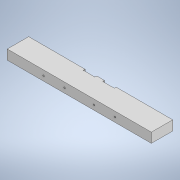
# Autodesk Inventor part: caster_wheel_mount
Saved by Autodesk Inventor 2020 (Build 240168000, 168)
## iProperties
Created: 2022-06-22
Part Number: caster_wheel_mount
Material: 일반
Document SubType Name: Modeling
Designer: samsung
Density: 1 g/cm^3
Appearance: 기본값
Author: samsung
Autodesk Inventor part; units mm, degrees
ref_plane "YZ Plane" through (0, 0, 0) normal (1, 0, 0) x (0, 1, 0)
ref_plane "작업 평면1" through (-15, 261.5, -15) normal (0, 1, 0) x (-1, 0, 0)
ref_plane "작업 평면4" through (-15, 241.5, -15) normal (0, 1, 0) x (1, 0, 0)
sketch "스케치4" plane through (-15, 241.5, -15) normal (0, 1, 0) x (1, 0, 0)
  line L0 (15, -15) -> (15, -10.3) projected
  line L1 (-15, -15) -> (15, -15) projected
  line L2 (-15, -10.3) -> (-15, -15) projected
  line L3 (-35, -10.3) -> (-15, -10.3) projected
  line L4 (-35, -15) -> (-35, -10.3) projected
  line L5 (-65, -15) -> (-35, -15) projected
  line L6 (-65, -10.3) -> (-65, -15) projected
  line L7 (-101.5, -10.3) -> (-65, -10.3) projected
  line L8 (51.5, -65.3) -> (-101.5, -65.3) projected
  line L9 (15, -10.3) -> (51.5, -10.3) projected
  line L10 (-105, -65.3) -> (-105, -10.3)
  line L11 (55, -65.3) -> (55, -10.3)
  line L12 (-105, -65.3) -> (55, -65.3)
  line L13 (-101.5, -10.3) -> (-65, -10.3) projected
  line L14 (-105, -10.3) -> (-65, -10.3)
  line L15 (55, -10.3) -> (15, -10.3)
  line L16 (15, -15) -> (15, -10.3) projected
  line L17 (15, -10.3) -> (15, -15)
  line L18 (15, -15) -> (13.8769, -15)
  line L19 (-65, -10.3) -> (-65, -15) projected
  line L20 (-65, -10.3) -> (-65, -15)
  line L21 (-65, -15) -> (-35, -15) projected
  line L22 (-65, -15) -> (-35, -15)
  line L23 (-35, -10.3) -> (-15, -10.3) projected
  line L24 (-35, -15) -> (-35, -10.3)
  line L25 (-15, -10.3) -> (-35, -10.3)
  line L26 (-15, -10.3) -> (-15, -15)
  line L27 (-15, -15) -> (15, -15) projected
  line L28 (-15, -15) -> (15, -15)
  line L29 (55, -65.3) -> (160.5, -65.3)
  line L30 (160.5, -65.3) -> (160.5, -10.3)
  line L31 (160.5, -10.3) -> (55, -10.3)
  line L32 (55, -10.3) -> (55, -65.3)
  line L33 (-105, -65.3) -> (-210.5, -65.3)
  line L34 (-210.5, -65.3) -> (-210.5, -10.3)
  line L35 (-210.5, -10.3) -> (-105, -10.3)
  line L36 (-105, -10.3) -> (-105, -65.3)
  dimension "d92" = 105.5
  dimension "d93" = 105.5
  constraints: 42 end point, 6 collinear, 4 parallel, 4 perpendicular, 3 vertical, 2 horizontal, 2 point on line
  measures "d92" distance of L31.end L30.end
  measures "d93" distance of L34.end L35.end
extrude "돌출3" add sketch "스케치4" against normal blind 25
sketch "스케치5" plane through (-120, 241.5, 50.3) normal (0, 0, 1) x (1, 0, 0)
  line L0 (0, 0) -> (160, 0) projected
  line L1 (80, -25) -> (80, 0)
  line L2 (-17.5, -25) -> (47.5, -25)
  line L3 (47.5, -25) -> (47.5, -1)
  line L4 (47.5, -1) -> (-17.5, -1)
  line L5 (-17.5, -1) -> (-17.5, -25)
  line L6 (-105.5, 0) -> (265.5, 0) projected
  line L7 (265.5, -25) -> (-105.5, -25) projected
  line L8 (112.5, -25) -> (177.5, -25)
  line L9 (177.5, -25) -> (177.5, -1)
  line L10 (177.5, -1) -> (112.5, -1)
  line L11 (112.5, -1) -> (112.5, -25)
  line L12 (15, -1) -> (15, -25)
  line L13 (145, -1) -> (145, -25)
  point P0 (120, -241.5)
  point P1 (-12, -13)
  point P2 (42, -13)
  point P3 (118, -13)
  point P4 (172, -13)
  dimension "d95" = 65
  dimension "d96" = 24
  dimension "d99" = 32.5
  dimension "d100" = 12
  dimension "d101" = 5.5
  dimension "d102" = 5.5
  dimension "d103" = 12
  dimension "d104" = 65
  dimension "d105" = 24
  dimension "d106" = 32.5
  dimension "d107" = 5.5
  dimension "d108" = 12
  dimension "d109" = 5.5
  dimension "d110" = 12
  constraints: 22 end point, 6 midpoint, 4 parallel, 2 horizontal, 2 perpendicular, 2 point on line, 1 vertical
  measures "d95" distance of L4.end L3.end
  measures "d96" distance of L3.end L2.end
  measures "d99" distance between parallel lines of L1 L3
  measures "d100" distance from line of L4 point (-12, -13)
  measures "d101" distance from line of L5 point (-12, -13)
  measures "d102" distance from line of point (42, -13) L3
  measures "d103" distance from line of point (42, -13) L4
  measures "d104" distance of L10.end L9.end
  measures "d105" distance of L9.end L8.end
  measures "d106" distance between parallel lines of L11 L1
  measures "d107" distance from line of L11 point (118, -13)
  measures "d108" distance from line of L10 point (118, -13)
  measures "d109" distance from line of L9 point (172, -13)
  measures "d110" distance from line of L10 point (172, -13)
hole "구멍1" at (-132, 228.5, 50.3) at (-78, 228.5, 50.3) at (-2, 228.5, 50.3) at (52, 228.5, 50.3) direction (0, 0, -1) diameter 4.134 depth 15 tip angle 118 thread size "M5x0.8" class "6H" standard "ISO Metric profile"
sketch "스케치6" plane through (-50, 241.5, 0) normal (0, 0, -1) x (-1, 0, 0)
  line L0 (0, 0) -> (30, 0) projected
  line L1 (0, 0) -> (0, -25) projected
  line L2 (30, -25) -> (0, -25) projected
  line L3 (30, 0) -> (30, -25) projected
  line L4 (-50, 0) -> (-20, 0) projected
  line L5 (-50, 0) -> (-50, -25) projected
  line L6 (-20, -25) -> (-50, -25) projected
  line L7 (-20, 0) -> (-20, -25) projected
  point P0 (-50, -241.5)
  point P1 (15, -15)
  point P2 (-35, -15)
  dimension "d54" = 15
  dimension "d56" = 15
  measures "d54" distance from line of point (15, -15) L0
  measures "d56" distance from line of L4 point (-35, -15)
hole "구멍2" at (-65, 226.5, 0) at (-15, 226.5, 0) direction (0, 0, 1) diameter 4.134 depth 15 tip angle 118 thread size "M5x0.8" class "6H" standard "ISO Metric profile"
sketch "스케치10" plane through (0, 216.5, -4.7) normal (0, 0, -1) x (-1, 0, 0)
  line L0 (0, 0) -> (-40, 0) projected
  line L1 (-40, 25) -> (0, 25) projected
  line L2 (-145.5, 0) -> (-120.5, 0)
  line L3 (-120.5, 0) -> (-120.5, 25)
  line L4 (-120.5, 25) -> (-145.5, 25)
  line L5 (-145.5, 25) -> (-145.5, 0)
  line L6 (80, 25) -> (120, 25) projected
  line L7 (225.5, 0) -> (200.5, 0)
  line L8 (200.5, 0) -> (200.5, 25)
  line L9 (200.5, 25) -> (225.5, 25)
  line L10 (225.5, 25) -> (225.5, 0)
  circle A0 centre (65, 10) radius 2.067 projected
  circle A1 centre (15, 10) radius 2.067 projected
  point P0 (0, -216.5)
  point P1 (213, 10)
  point P2 (-133, 10)
  dimension "d69" = 25
  dimension "d70" = 25
  dimension "d71" = 12.5
  dimension "d72" = 12.5
  constraints: 16 end point, 4 parallel, 3 point on line, 2 horizontal, 2 horizontal alignment, 2 perpendicular
  measures "d69" distance of L4.end L3.end
  measures "d70" distance of L9.end L8.end
  measures "d71" distance from line of L10 point (213, 10)
  measures "d72" distance from line of L5 point (-133, 10)
hole "구멍3" at (-213, 226.5, -4.7) at (133, 226.5, -4.7) direction (0, 0, 1) diameter 4.134 depth 15 tip angle 118 thread size "M5x0.8" class "6H" standard "ISO Metric profile"
